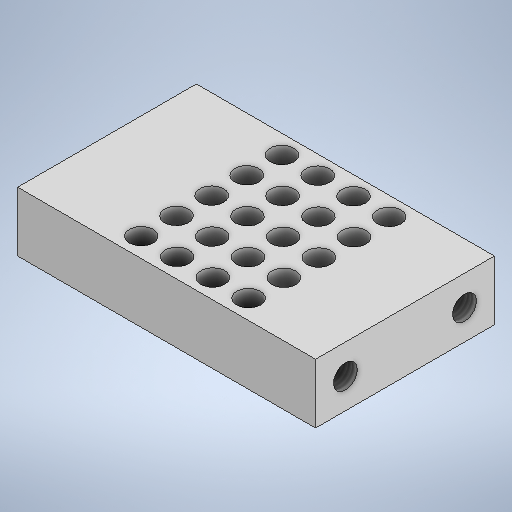
# Autodesk Inventor part: cubito pro max
Saved by Autodesk Inventor 2025.2 (Build 292293000, 293)
## iProperties
Created: 2025-04-07
Part Number: cubito pro max
Material: Generic
Document SubType Name: Modeling
Designer: maqmat
Density: 1 g/cm^3
Appearance: Default
Author: maqmat
Autodesk Inventor part; units mm, degrees
ref_plane "YZ Plane" through (0, 0, 0) normal (1, 0, 0) x (0, 1, 0)
ref_plane "XZ Plane" through (0, 0, 0) normal (0, 1, 0) x (-1, 0, 0)
ref_plane "XY Plane" through (0, 0, 0) normal (0, 0, 1) x (1, 0, 0)
sketch "Sketch1" plane through (0, 0, 0) normal (0, 1, 0) x (-1, 0, 0)
  line L0 (-4.0944, 5.5957) -> (45.9056, 5.5957)
  line L1 (45.9056, 5.5957) -> (45.9056, -24.4043)
  line L2 (45.9056, -24.4043) -> (-4.0944, -24.4043)
  line L3 (-4.0944, -24.4043) -> (-4.0944, 5.5957)
  point P0 (0, 0)
  dimension "d0" = 50
  dimension "d1" = 30
  constraints: 8 end point, 2 parallel, 1 horizontal, 1 perpendicular
  measures "d0" distance of L1.end L2.end
  measures "d1" distance of L0.end L1.end
extrude "Extrusion1" add sketch "Sketch1" along normal blind 10
sketch "Sketch2" plane through (4.0944, 0, 5.5957) normal (1, 0, 0) x (0, 0, -1)
  line L0 (30, 0) -> (0, 0) projected
  line L1 (15, 0) -> (15, 10)
  line L2 (30, 10) -> (0, 10) projected
  line L3 (15, 5) -> (5, 5)
  line L4 (15, 5) -> (25, 5)
  circle A0 centre (5, 5) radius 2
  circle A1 centre (25, 5) radius 2
  point P0 (5.5957, 0)
  dimension "d4" = 10
  dimension "d5" = 10
  dimension "d6" = 4
  dimension "d7" = 4
  constraints: 6 end point, 3 midpoint, 2 centre point, 2 coincident, 1 horizontal, 1 point on line
  measures "d4" distance of L3.start L3.end
  measures "d5" distance of L3.start L4.end
  measures "d6" diameter of A0
  measures "d7" diameter of A1
extrude "Extrusion2" cut sketch "Sketch2" against normal blind 10
sketch "Sketch3" plane through (-45.9056, 0, -24.4043) normal (-1, 0, 0) x (0, 0, 1)
  line L0 (30, 0) -> (0, 0) projected
  line L1 (15, 0) -> (15, 10)
  line L2 (30, 10) -> (0, 10) projected
  line L3 (15, 5) -> (5, 5)
  line L4 (15, 5) -> (25, 5)
  circle A0 centre (5, 5) radius 2 projected
  circle A1 centre (5, 5) radius 2
  circle A2 centre (25, 5) radius 2 projected
  circle A3 centre (25, 5) radius 2
  point P0 (24.4043, 0)
  dimension "d10" = 10
  dimension "d11" = 10
  constraints: 6 end point, 3 midpoint, 2 centre point, 2 coincident, 2 horizontal
  measures "d10" distance of L3.start L3.end
  measures "d11" distance of L3.start L4.end
extrude "Extrusion3" cut sketch "Sketch3" against normal blind 10
sketch "Sketch4" plane through (0, 10, 0) normal (0, 1, 0) x (1, 0, 0)
  line L0 (-45.9056, 24.4043) -> (-45.9056, -5.5957) projected
  line L1 (-45.9056, 9.4043) -> (4.0944, 9.4043)
  line L2 (4.0944, -5.5957) -> (4.0944, 24.4043) projected
  line L3 (-20.9056, 9.4043) -> (-20.9056, -5.5957)
  line L4 (-45.9056, -5.5957) -> (4.0944, -5.5957) projected
  line L5 (-20.9056, 9.4043) -> (-20.9056, 24.4043)
  line L6 (-20.9056, 16.9043) -> (-35.9056, 16.9043)
  line L7 (-45.9056, 17.4043) -> (-35.9056, 17.4043) projected
  line L8 (-20.9056, 16.9043) -> (-5.9056, 16.9043)
  line L9 (-5.9056, 1.4043) -> (-5.9056, -2.5957) projected
  line L10 (-20.9056, 1.4043) -> (-5.9056, 1.4043)
  line L11 (-20.9056, 1.4043) -> (-35.9056, 1.4043)
  line L12 (-28.4056, 16.9043) -> (-28.4056, -5.5957)
  line L13 (-28.4056, 24.4043) -> (-28.4056, -5.5957)
  line L14 (-28.4056, 16.9043) -> (-20.9056, 16.9043)
  line L15 (-20.9056, 9.4043) -> (-28.4056, 9.4043)
  line L16 (-20.9056, 1.4043) -> (-28.4056, 1.4043)
  line L17 (-20.9056, 0) -> (-28.4056, 0)
  circle A0 centre (-28.4056, 21.2599) radius 2
  circle A1 centre (-28.4056, 21.2599) radius 2
  circle A2 centre (-28.4056, 15.3599) radius 2
  circle A3 centre (-28.4056, 9.4599) radius 2
  circle A4 centre (-28.4056, 3.5599) radius 2
  circle A5 centre (-28.4056, -2.3401) radius 2
  circle A6 centre (-22.4056, 21.2599) radius 2
  circle A7 centre (-22.4056, 15.3599) radius 2
  circle A8 centre (-22.4056, 9.4599) radius 2
  circle A9 centre (-22.4056, 3.5599) radius 2
  circle A10 centre (-22.4056, -2.3401) radius 2
  circle A11 centre (-16.4056, 21.2599) radius 2
  circle A12 centre (-16.4056, 15.3599) radius 2
  circle A13 centre (-16.4056, 9.4599) radius 2
  circle A14 centre (-16.4056, 3.5599) radius 2
  circle A15 centre (-16.4056, -2.3401) radius 2
  circle A16 centre (-10.4056, 21.2599) radius 2
  circle A17 centre (-10.4056, 15.3599) radius 2
  circle A18 centre (-10.4056, 9.4599) radius 2
  circle A19 centre (-10.4056, 3.5599) radius 2
  circle A20 centre (-10.4056, -2.3401) radius 2
  point P0 (0, 0)
  dimension "d17" = 4
  dimension "d27" = 5.9
  dimension "d30" = 6
  constraints: 26 end point, 21 centre point, 9 point on line, 8 midpoint, 3 collinear, 2 coincident, 2 parallel, 2 perpendicular, 2 vertical, 1 horizontal, 38 other
  measures "d17" diameter of A0
  measures "d27" distance of A0.centre A2.centre
  measures "d30" distance of A0.centre A6.centre
extrude "Extrusion4" cut sketch "Sketch4" against normal blind 10 contours A0 L13 | L13 A0 | A6 L5 | L5 A6 | A17 L8 | L8 A17 | A12 L8 | L8 A12 | A3 L12 L1 | L1 L12 A3 | L12 A3 L1 | L1 A3 L12 | A5 L12 | L12 A5 | A2 L6 L12 | L12 L6 A2 | A4 L12 | L12 A4 | A10 L3 | L3 A10 | A8 L5 L1 | L1 L3 A8 | L13 A2 L6 | L6 A2 L13 | L5 A8 L1 | L1 A8 L3 | A18 L1 | L1 A18 | A7 L6 L5 | L5 A7 | A9 L3 | L3 A9 | A7 L6 | A13 L1 | L1 A13 | A11 | A14 | A15 | A16 | A19 | A20 picked at (-21.946, 15.7701)
thread "Thread1" size "M4x0.7" class "6H" standard "ANSI Metric M Profile" full length
thread "Thread2" size "M4x0.7" class "6H" standard "ANSI Metric M Profile" full length
thread "Thread3" size "M4x0.7" class "6H" standard "ANSI Metric M Profile" full length
thread "Thread4" size "M4x0.7" class "6H" standard "ANSI Metric M Profile" full length
body "Solid1"
